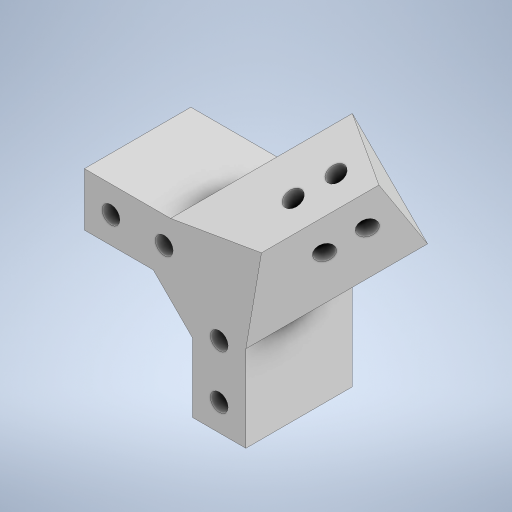
# Autodesk Inventor part: EX-L-Connect
Saved by Autodesk Inventor 2024.3 (Build 283343000, 343)
## iProperties
Created: 2025-11-26
Part Number: EX-L-Connect
Material: 一般
Document SubType Name: Modeling
Designer: 佐藤智貴
Density: 1 g/cm^3
Appearance: 既定
Author: 佐藤智貴
Autodesk Inventor part; units mm, degrees
ref_plane "YZ Plane" through (0, 0, 0) normal (1, 0, 0) x (0, 1, 0)
ref_plane "XZ Plane" through (0, 0, 0) normal (0, 1, 0) x (-1, 0, 0)
ref_plane "XY Plane" through (0, 0, 0) normal (0, 0, 1) x (1, 0, 0)
sketch "スケッチ1" plane through (0, 0, 0) normal (0, 0, 1) x (1, 0, 0)
  line L0 (0, 0) -> (60, 0)
  line L1 (60, 0) -> (60, 60)
  line L2 (60, 60) -> (0, 60)
  line L3 (0, 60) -> (0, 0)
  dimension "d0" = 60
  dimension "d1" = 60
  constraints: 8 end point, 2 parallel, 1 horizontal, 1 perpendicular
  measures "d0" distance of L1.end L2.end
  measures "d1" distance of L0.end L1.end
extrude "押し出し1" add sketch "スケッチ1" along normal blind 30
sketch "スケッチ2" plane through (0, 0, 30) normal (0, 0, 1) x (1, 0, 0)
  line L0 (60, 0) -> (60, 60) projected
  line L1 (60, 60) -> (0, 60) projected
  point P0 (0, 0)
  point P1 (22, 49.5)
  point P2 (37, 49.5)
  point P3 (52.5, 34)
  point P4 (52.5, 19)
  dimension "d4" = 7.5
  dimension "d5" = 7.5
  dimension "d6" = 10.5
  dimension "d7" = 10.5
  dimension "d8" = 15
  dimension "d9" = 15
  dimension "d10" = 23
  dimension "d11" = 26
  measures "d4" distance from line of L0 point (52.5, 34)
  measures "d5" distance from line of L0 point (52.5, 19)
  measures "d6" distance from line of L1 point (37, 49.5)
  measures "d7" distance from line of L1 point (22, 49.5)
  measures "d8" distance of point (22, 49.5) point (37, 49.5)
  measures "d9" distance of point (52.5, 19) point (52.5, 34)
  measures "d10" distance from line of L0 point (37, 49.5)
  measures "d11" distance from line of L1 point (52.5, 34)
hole "穴1" at (22, 49.5, 30) at (37, 49.5, 30) at (52.5, 34, 30) at (52.5, 19, 30) direction (0, 0, -1) diameter 5 end through all
sketch "スケッチ3" plane through (0, 0, 30) normal (0, 0, 1) x (1, 0, 0)
  line L0 (22, 49.5) -> (37, 49.5)
  circle A0 centre (52.5, 34) radius 2.5 projected
  line L1 (37, 49.5) -> (52.5, 34)
  line L2 (52.5, 34) -> (52.5, 19)
  line L3 (22, 49.5) -> (22, 19)
  line L4 (22, 19) -> (52.5, 19)
  line L5 (60, 37.1066) -> (40.1066, 57)
  line L6 (40.1066, 57) -> (14.5, 57)
  line L7 (14.5, 57) -> (14.5, 11.5)
  line L8 (14.5, 11.5) -> (60, 11.5)
  line L9 (60, 11.5) -> (60, 37.1066)
  line L10 (14.5, 57) -> (44.5, 57)
  line L11 (44.5, 57) -> (44.5, 42)
  line L12 (44.5, 42) -> (14.5, 42)
  line L13 (14.5, 42) -> (14.5, 57)
  line L14 (60, 11.5) -> (45, 11.5)
  line L15 (45, 11.5) -> (45, 41.5)
  line L16 (45, 41.5) -> (60, 41.5)
  line L17 (60, 41.5) -> (60, 11.5)
  circle A1 centre (52.5, 19) radius 2.5 projected
  circle A2 centre (52.5, 34) radius 2.5 projected
  circle A3 centre (37, 49.5) radius 2.5 projected
  circle A4 centre (22, 49.5) radius 2.5 projected
  line L18 (60, 0) -> (60, 60) projected
  line L19 (60, 60) -> (0, 60) projected
  line L20 (0, 60) -> (0, 0) projected
  line L21 (0, 0) -> (60, 0) projected
  line L22 (14.5, 42) -> (45, 11.5)
  line L23 (24.0029, 51.8905) -> (54.5029, 21.3905)
  line L24 (38.7868, 57) -> (60, 35.7868)
  point P0 (52.5, 26.5)
  point P1 (45, 19)
  point P2 (22, 42)
  point P3 (39.2529, 36.6405)
  point P4 (45, 30.8934)
  point P5 (33.8934, 42)
  dimension "d19" = 7.5
  dimension "d20" = 7.5
  dimension "d21" = 7.5
  dimension "d22" = 30
  dimension "d23" = 30
  dimension "d50" = 7.5
  dimension "d52" = 30
  constraints: 42 end point, 6 parallel, 6 perpendicular, 3 horizontal, 2 midpoint, 2 point on line, 1 vertical, 4 other
  measures "d19" distance between parallel lines of L0 L6
  measures "d20" distance between parallel lines of L0 L12
  measures "d21" distance from line of point (52.5, 26.5) L15
  measures "d22" distance between parallel lines of L13 L11
  measures "d23" distance between parallel lines of L14 L16
  measures "d50" distance from line of L1 point (39.253, 36.64)
  measures "d52" distance of L24.start L24.end
extrude "押し出し2" cut sketch "スケッチ3" against normal blind 30 contours L12 L23 L15 L4 L22 L3 | L3 L22 L12 | L22 L4 L3 | L3 L4 L22 L8 L7 | L7 L8 L18 L21 L20 L19 L16 L5 L11 L10 L6 | L4 L15 L22 | L24 L6 L5 L11 | L11 L5 L16 L24 | L16 L5 L9 L24 | L5 L10 L11 | L16 L17 L5
sketch "スケッチ15" plane through (60, 35.7868, 0) normal (0.7071068, 0.7071068, 0) x (-0.7071068, 0.7071068, 0)
  line L0 (0, 30) -> (30, 30) projected
  line L1 (0, 0) -> (0, 30) projected
  line L2 (30, 0) -> (0, 0) projected
  line L3 (30, 30) -> (30, 0) projected
  point P0 (17.1213, 0)
extrude "押し出し11" add sketch "スケッチ15" along normal blind 30
sketch "スケッチ16" plane through (60, 35.7868, 30) normal (0.7071068, -0.7071068, 0) x (-0.7071068, -0.7071068, 0)
  line L0 (0, 30) -> (0, 0) projected
  line L1 (0, 30) -> (-30, 30) projected
  line L2 (-30, 0) -> (-30, 30) projected
  line L3 (0, 0) -> (-30, 0) projected
  line L4 (0, 0) -> (-30, 30)
  point P0 (67.7315, 30)
  constraints: 2 end point
extrude "押し出し12" cut sketch "スケッチ16" against normal blind 30 contours L3 L2 L4
sketch "スケッチ18" plane through (60, 35.7868, 30) normal (0.5, 0.5, 0.7071068) x (0.7071068, -0.7071068, 0)
  line L0 (0, 42.4264) -> (0, 0) projected
  line L1 (0, 42.4264) -> (-30, 42.4264) projected
  line L2 (-30, 0) -> (-30, 42.4264) projected
  line L3 (0, 0) -> (-30, 0) projected
  point P0 (-17.1213, -26.6802)
extrude "押し出し13" add sketch "スケッチ18" along normal blind 30
sketch "スケッチ19" plane through (81.2132, 57, 0) normal (0.5, 0.5, -0.7071068) x (-0.5, -0.5, -0.7071068)
  line L0 (21.2132, 0) -> (0, 0) projected
  line L1 (0, 30) -> (-30, 30) projected
  line L2 (0, 0) -> (-30, 30)
  line L3 (-30, 30) -> (0, 30)
  line L4 (0, 0) -> (-30, 0) projected
  line L5 (0, 30) -> (-30, 0)
  line L6 (0, 0) -> (0, 30) projected
  line L7 (0, 30) -> (-30, 30) projected
  line L8 (-30, 0) -> (-30, 30) projected
  line L9 (0, 0) -> (-30, 0) projected
  point P0 (69.1066, 17.1213)
  point P1 (-15, 15)
  constraints: 6 end point, 1 collinear, 1 perpendicular
extrude "押し出し14" cut sketch "スケッチ19" against normal through all contours L5 L2 L1 | L2 L5 L8 | L2 L4 L5
sketch "スケッチ20" plane through (0, 0, 30) normal (0, 0, 1) x (1, 0, 0)
  circle A0 centre (52.5, 19) radius 2.5 projected
  circle A1 centre (52.5, 34) radius 2.5 projected
  circle A2 centre (37, 49.5) radius 2.5 projected
  circle A3 centre (22, 49.5) radius 2.5 projected
  line L0 (60, 35.7868) -> (38.7868, 57) projected
  line L1 (38.7868, 57) -> (14.5, 57) projected
  line L2 (14.5, 57) -> (14.5, 42) projected
  line L3 (14.5, 42) -> (33.8934, 42) projected
  line L4 (33.8934, 42) -> (45, 30.8934) projected
  line L5 (45, 30.8934) -> (45, 11.5) projected
  line L6 (45, 11.5) -> (60, 11.5) projected
  line L7 (60, 11.5) -> (60, 35.7868) projected
  line L8 (38.7868, 57) -> (60, 78.2132) projected
  line L9 (38.7868, 57) -> (60, 78.2132)
  line L10 (60, 78.2132) -> (81.2132, 57)
  line L11 (81.2132, 57) -> (60, 35.7868)
  point P0 (0, 0)
  constraints: 6 end point, 2 perpendicular, 1 collinear
extrude "押し出し15" cut sketch "スケッチ20" along normal blind 15 contours L0 L8 L10 L11
sketch "スケッチ23" plane through (81.2132, 57, 0) normal (0.8535534, -0.1464466, 0.5) x (0.5, 0.5, -0.7071068)
  line L0 (0, 21.2132) -> (0, 0) projected
  line L1 (-27.4264, 21.2132) -> (-42.4264, 0) projected
  line L2 (0, 0) -> (-27.4264, 0)
  line L3 (-27.4264, 0) -> (-27.4264, 21.2132)
  line L4 (-27.4264, 21.2132) -> (0, 21.2132)
  line L5 (0, 21.2132) -> (0, 0)
  point P0 (-69.1066, -36.7591)
  point P1 (-17.4264, 12.4132)
  point P2 (-7.4264, 12.4132)
  dimension "d71" = 10
  dimension "d72" = 10
  dimension "d93" = 8.8
  dimension "d94" = 8.8
  constraints: 8 end point, 2 parallel, 1 horizontal, 1 perpendicular
  measures "d71" distance from line of L3 point (-17.426, 12.413)
  measures "d72" distance of point (-7.426, 12.413) point (-17.426, 12.413)
  measures "d93" distance from line of L4 point (-17.426, 12.413)
  measures "d94" distance from line of L4 point (-7.426, 12.413)
hole "穴2" at (70.6821, 58.8821, 18.5289) at (75.6821, 63.8821, 11.4579) direction (-0.8535534, 0.1464466, -0.5) diameter 5 depth 8
sketch "スケッチ24" plane through (60, 78.2132, 0) normal (-0.1464466, 0.8535534, 0.5) x (0.8535534, -0.1464466, 0.5)
  line L0 (21.2132, -27.4264) -> (21.2132, -42.4264) projected
  line L1 (-15, -21.2132) -> (0, 0) projected
  line L2 (21.2132, -27.4264) -> (0, -27.4264)
  line L3 (0, -27.4264) -> (0, 0)
  line L4 (0, 0) -> (21.2132, 0)
  line L5 (21.2132, 0) -> (21.2132, -27.4264)
  point P0 (-39.7591, -69.1066)
  point P1 (12.4132, -17.4264)
  point P2 (12.4132, -7.4264)
  dimension "d82" = 10
  dimension "d83" = 10
  dimension "d95" = 8.8
  dimension "d96" = 8.8
  constraints: 8 end point, 2 parallel, 1 horizontal, 1 perpendicular
  measures "d82" distance from line of L2 point (12.413, -17.426)
  measures "d83" distance of point (12.413, -7.426) point (12.413, -17.426)
  measures "d95" distance from line of L5 point (12.413, -17.426)
  measures "d96" distance from line of L5 point (12.413, -7.426)
hole "穴3" at (61.8821, 67.6821, 18.5289) at (66.8821, 72.6821, 11.4579) direction (0.1464466, -0.8535534, -0.5) diameter 5 depth 8
equation "\"d5\" = d4"
equation "\"d7\" = d6"
equation "\"d9\" = d8"
equation "\"d20\" = d19"
equation "\"d21\" = d20"
equation "\"d23\" = d22"
equation "\"d94\" = d93"
equation "\"d83\" = d82"
equation "\"d96\" = d95"
